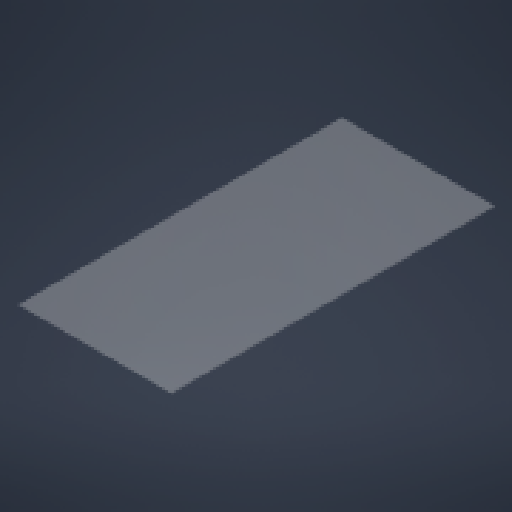
# Autodesk Inventor part: polycarb10x6
Saved by Autodesk Inventor 2023 (Build 270158000, 158)
## iProperties
Created: 2023-01-26
Part Number: polycarb10x6
Material: Polycarbonate, Clear
Document SubType Name: Modeling
Designer: Windows Macbook
Density: 1.2 g/cm^3
Appearance: Polycarbonate - Clear
Author: Windows Macbook
Autodesk Inventor part; units mm, degrees
ref_plane "YZ Plane" through (0, 0, 0) normal (1, 0, 0) x (0, 1, 0)
ref_plane "XZ Plane" through (0, 0, 0) normal (0, 1, 0) x (-1, 0, 0)
ref_plane "XY Plane" through (0, 0, 0) normal (0, 0, 1) x (1, 0, 0)
sketch "Sketch1" plane through (0, 0, 0) normal (0, 1, 0) x (-1, 0, 0)
  line L0 (-101.6, -195.8975) -> (50.8, -195.8975)
  line L1 (50.8, -195.8975) -> (50.8, 127)
  line L2 (50.8, 127) -> (-101.6, 127)
  line L3 (-101.6, 127) -> (-101.6, -195.8975)
  point P0 (0, 0)
  dimension "d0" = 152.4
  dimension "d1" = 322.8975
  constraints: 8 end point, 2 parallel, 1 horizontal, 1 perpendicular
  measures "d0" distance of L2.end L1.end
  measures "d1" distance of L1.end L0.end
extrude "Extrusion2" add sketch "Sketch1" along normal blind 1.5875
sketch "Sketch2" plane through (0, 0, 0) normal (1, 0, 0) x (0, 1, 0)
  line L0 (1.5875, -195.8975) -> (1.5875, 127) projected
  line L1 (1.5875, 127) -> (0, 125.4125)
  line L2 (0, -195.8975) -> (0, 127) projected
  line L3 (1.5875, 127) -> (3.8326, 127) construction
  line L4 (1.5875, 127) -> (0, 127)
  line L5 (0, 127) -> (0, 125.4125)
  point P0 (0, 0)
  dimension "d8" = 135
  constraints: 8 end point, 2 horizontal, 1 collinear, 1 equal length, 1 point on line
  measures "d8" angle of L1 L3
extrude "Extrusion3" cut sketch "Sketch2" along normal blind 203.2 and the other way blind 152.4
body "Solid2"
